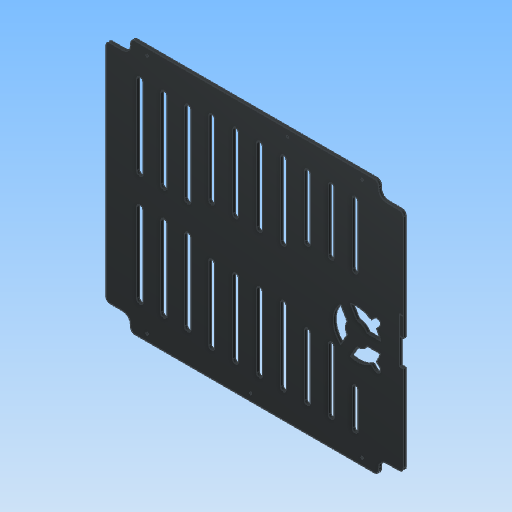
# Autodesk Inventor part: поддон1
Saved by Autodesk Inventor 2017 (Build 210142000, 142)
## iProperties
Part Number: поддон1
Material: Типовые
Document SubType Name: Modeling
Designer: Max
Density: 1 g/cm^3
Appearance: Чугун серый
Mass: 323.562 g
Surface Area: 2205.86 cm^2
Volume: 323.562 cm^3
Author: Max
Autodesk Inventor part; units mm, degrees
ref_plane "YZ Plane" through (0, 0, 0) normal (1, 0, 0) x (0, 1, 0)
ref_plane "XZ Plane" through (0, 0, 0) normal (0, 1, 0) x (-1, 0, 0)
ref_plane "XY Plane" through (0, 0, 0) normal (0, 0, 1) x (1, 0, 0)
sketch "Эскиз1" plane through (0, 0, 0) normal (0, 0, 1) x (1, 0, 0)
  line L0 (186.5, -159.5) -> (-186.5, -159.5)
  line L1 (-186.5, -159.5) -> (-186.5, 159.5)
  line L2 (-186.5, 159.5) -> (186.5, 159.5)
  line L3 (186.5, 159.5) -> (186.5, -159.5)
  line L4 (186.5, -159.5) -> (-186.5, 159.5) construction
  line L5 (-186.5, -159.5) -> (186.5, 159.5) construction
  circle A0 centre (-2.4493, 121.4084) radius 1.5 construction
  circle A1 centre (336.5507, 121.4084) radius 1.5 construction
  circle A2 centre (336.5507, 427.4084) radius 1.5 construction
  circle A3 centre (-2.4493, 427.4084) radius 1.5 construction
  arc A4 (348.5507, 300.4084) -> (346.5507, 298.4084) centre (348.5507, 298.4084) ccw construction
  line L6 (348.5507, 300.4084) -> (350.5507, 300.4084) construction
  arc A5 (350.5507, 300.4084) -> (350.5507, 305.4084) centre (350.5507, 302.9084) ccw construction
  line L7 (350.5507, 305.4084) -> (348.5507, 305.4084) construction
  arc A6 (346.5507, 307.4084) -> (348.5507, 305.4084) centre (348.5507, 307.4084) ccw construction
  line L8 (346.5507, 307.4084) -> (346.5507, 412.4084) construction
  line L9 (346.5507, 412.4084) -> (267.5507, 412.4084) construction
  arc A7 (265.5507, 414.4084) -> (267.5507, 412.4084) centre (267.5507, 414.4084) ccw construction
  line L10 (265.5507, 414.4084) -> (265.5507, 416.4084) construction
  arc A8 (265.5507, 416.4084) -> (250.5507, 416.4084) centre (258.0507, 416.4084) ccw construction
  line L11 (250.5507, 416.4084) -> (250.5507, 414.4084) construction
  arc A9 (248.5507, 412.4084) -> (250.5507, 414.4084) centre (248.5507, 414.4084) ccw construction
  line L12 (248.5507, 412.4084) -> (192.5507, 412.4084) construction
  arc A10 (190.5507, 414.4084) -> (192.5507, 412.4084) centre (192.5507, 414.4084) ccw construction
  line L13 (190.5507, 414.4084) -> (190.5507, 421.9084) construction
  arc A11 (190.5507, 421.9084) -> (188.5507, 423.9084) centre (188.5507, 421.9084) ccw construction
  line L14 (188.5507, 423.9084) -> (142.5507, 423.9084) construction
  arc A12 (142.5507, 423.9084) -> (140.5507, 421.9084) centre (142.5507, 421.9084) ccw construction
  line L15 (140.5507, 421.9084) -> (140.5507, 414.4084) construction
  arc A13 (138.5507, 412.4084) -> (140.5507, 414.4084) centre (138.5507, 414.4084) ccw construction
  line L16 (138.5507, 412.4084) -> (82.5507, 412.4084) construction
  arc A14 (80.5507, 414.4084) -> (82.5507, 412.4084) centre (82.5507, 414.4084) ccw construction
  line L17 (80.5507, 414.4084) -> (80.5507, 416.4084) construction
  arc A15 (80.5507, 416.4084) -> (65.5507, 416.4084) centre (73.0507, 416.4084) ccw construction
  line L18 (65.5507, 416.4084) -> (65.5507, 414.4084) construction
  arc A16 (63.5507, 412.4084) -> (65.5507, 414.4084) centre (63.5507, 414.4084) ccw construction
  line L19 (63.5507, 412.4084) -> (-15.4493, 412.4084) construction
  line L20 (-15.4493, 412.4084) -> (-15.4493, 136.4084) construction
  line L21 (-15.4493, 136.4084) -> (92.5507, 136.4084) construction
  arc A17 (94.5507, 134.4084) -> (92.5507, 136.4084) centre (92.5507, 134.4084) ccw construction
  line L22 (94.5507, 134.4084) -> (94.5507, 122.4084) construction
  arc A18 (94.5507, 122.4084) -> (96.5507, 120.4084) centre (96.5507, 122.4084) ccw construction
  line L23 (96.5507, 120.4084) -> (127.5507, 120.4084) construction
  arc A19 (127.5507, 120.4084) -> (129.5507, 122.4084) centre (127.5507, 122.4084) ccw construction
  line L24 (129.5507, 122.4084) -> (129.5507, 134.4084) construction
  arc A20 (131.5507, 136.4084) -> (129.5507, 134.4084) centre (131.5507, 134.4084) ccw construction
  line L25 (131.5507, 136.4084) -> (164.5507, 136.4084) construction
  arc A21 (166.5507, 134.4084) -> (164.5507, 136.4084) centre (164.5507, 134.4084) ccw construction
  line L26 (166.5507, 134.4084) -> (166.5507, 119.4084) construction
  arc A22 (166.5507, 119.4084) -> (168.5507, 117.4084) centre (168.5507, 119.4084) ccw construction
  line L27 (168.5507, 117.4084) -> (289.5507, 117.4084) construction
  arc A23 (289.5507, 117.4084) -> (291.5507, 119.4084) centre (289.5507, 119.4084) ccw construction
  line L28 (291.5507, 119.4084) -> (291.5507, 134.4084) construction
  arc A24 (293.5507, 136.4084) -> (291.5507, 134.4084) centre (293.5507, 134.4084) ccw construction
  line L29 (293.5507, 136.4084) -> (346.5507, 136.4084) construction
  line L30 (346.5507, 136.4084) -> (346.5507, 196.4084) construction
  arc A25 (348.5507, 198.4084) -> (346.5507, 196.4084) centre (348.5507, 196.4084) ccw construction
  line L31 (348.5507, 198.4084) -> (350.5507, 198.4084) construction
  arc A26 (350.5507, 198.4084) -> (350.5507, 203.4084) centre (350.5507, 200.9084) ccw construction
  line L32 (350.5507, 203.4084) -> (348.5507, 203.4084) construction
  arc A27 (346.5507, 205.4084) -> (348.5507, 203.4084) centre (348.5507, 205.4084) ccw construction
  line L33 (346.5507, 205.4084) -> (346.5507, 298.4084) construction
  circle A28 centre (208.5507, 425.4084) radius 1.5 construction
  circle A29 centre (302.0507, 425.4084) radius 1.5 construction
  circle A30 centre (162.0507, 123.4084) radius 1.5 construction
  circle A31 centre (-2.4493, 427.4084) radius 1.5 construction
  circle A32 centre (336.5507, 121.4084) radius 1.5 construction
  circle A33 centre (351.5507, 272.4084) radius 1.5 construction
  circle A34 centre (351.5507, 252.4084) radius 1.5 construction
  circle A35 centre (-2.4493, 121.4084) radius 1.5 construction
  circle A36 centre (336.5507, 427.4084) radius 1.5 construction
  circle A37 centre (32.5507, 123.4084) radius 1.5 construction
  circle A38 centre (302.0507, 123.4084) radius 1.5 construction
  circle A39 centre (32.5507, 425.4084) radius 1.5 construction
  line L34 (-23.4493, 108.4084) -> (354.5507, 108.4084) construction
  line L35 (-23.4493, 440.4084) -> (-23.4493, 108.4084) construction
  line L36 (354.5507, 440.4084) -> (-23.4493, 440.4084) construction
  line L37 (354.5507, 108.4084) -> (354.5507, 440.4084) construction
  line L38 (134.75, 151) -> (-134.75, 151) construction
  line L39 (-134.75, 151) -> (-134.75, -151) construction
  line L40 (-134.75, -151) -> (134.75, -151) construction
  line L41 (134.75, -151) -> (134.75, 151) construction
  line L42 (134.75, 151) -> (-134.75, -151) construction
  line L43 (-134.75, 151) -> (134.75, -151) construction
  circle A40 centre (-134.75, -151) radius 1.5
  circle A41 centre (134.75, -151) radius 1.5
  circle A42 centre (134.75, 151) radius 1.5
  circle A43 centre (-134.75, 151) radius 1.5
  point P0 (0, 0)
  dimension "d0" = 373
  dimension "d1" = 319
  dimension "d2" = 3
  dimension "d3" = 3
  dimension "d4" = 3
  dimension "d5" = 3
  dimension "d6" = 8.5
  dimension "d7" = 8.5
  dimension "d8" = 51.75
  dimension "d11" = 269.5
  dimension "d12" = 302
  constraints: 24 end point, 4 centre point, 4 coincident, 4 midpoint, 4 parallel, 2 horizontal, 2 perpendicular
  measures "d0" distance between parallel lines of L1 L3
  measures "d1" distance between parallel lines of L0 L2
  measures "d2" diameter of A40
  measures "d3" diameter of A41
  measures "d4" diameter of A42
  measures "d5" diameter of A43
  measures "d6" distance from line of L2 L38.end
  measures "d7" distance from line of L0 L39.end
  measures "d8" distance between parallel lines of L1 L39
  measures "d11" distance of L38.end L38.start
  measures "d12" distance between parallel lines of L38 L40
extrude "Выдавливание1" add sketch "Эскиз1" along normal blind 3.2
sketch "Эскиз2" plane through (0, 0, 0) normal (0, 0, -1) x (-1, 0, 0)
  arc A0 (-179.25, 24) -> (-181.25, 26) centre (-181.25, 24) ccw projected
  line L0 (-181.25, 26) -> (-183.25, 26) projected
  arc A1 (-183.25, 31) -> (-183.25, 26) centre (-183.25, 28.5) ccw projected
  line L1 (-183.25, 31) -> (-181.25, 31) projected
  arc A2 (-181.25, 31) -> (-179.25, 33) centre (-181.25, 33) ccw projected
  line L2 (-179.25, 33) -> (-179.25, 138) projected
  line L3 (-179.25, 138) -> (-100.25, 138) projected
  arc A3 (-100.25, 138) -> (-98.25, 140) centre (-100.25, 140) ccw projected
  line L4 (-98.25, 140) -> (-98.25, 142) projected
  arc A4 (-83.25, 142) -> (-98.25, 142) centre (-90.75, 142) ccw projected
  line L5 (-83.25, 142) -> (-83.25, 140) projected
  arc A5 (-83.25, 140) -> (-81.25, 138) centre (-81.25, 140) ccw projected
  line L6 (-81.25, 138) -> (-25.25, 138) projected
  arc A6 (-25.25, 138) -> (-23.25, 140) centre (-25.25, 140) ccw projected
  line L7 (-23.25, 140) -> (-23.25, 147.5) projected
  arc A7 (-21.25, 149.5) -> (-23.25, 147.5) centre (-21.25, 147.5) ccw projected
  line L8 (-21.25, 149.5) -> (24.75, 149.5) projected
  arc A8 (26.75, 147.5) -> (24.75, 149.5) centre (24.75, 147.5) ccw projected
  line L9 (26.75, 147.5) -> (26.75, 140) projected
  arc A9 (26.75, 140) -> (28.75, 138) centre (28.75, 140) ccw projected
  line L10 (28.75, 138) -> (84.75, 138) projected
  arc A10 (84.75, 138) -> (86.75, 140) centre (84.75, 140) ccw projected
  line L11 (86.75, 140) -> (86.75, 142) projected
  arc A11 (101.75, 142) -> (86.75, 142) centre (94.25, 142) ccw projected
  line L12 (101.75, 142) -> (101.75, 140) projected
  arc A12 (101.75, 140) -> (103.75, 138) centre (103.75, 140) ccw projected
  line L13 (103.75, 138) -> (182.75, 138) projected
  line L14 (182.75, 138) -> (182.75, -138) projected
  line L15 (182.75, -138) -> (74.75, -138) projected
  arc A13 (74.75, -138) -> (72.75, -140) centre (74.75, -140) ccw projected
  line L16 (72.75, -140) -> (72.75, -152) projected
  arc A14 (70.75, -154) -> (72.75, -152) centre (70.75, -152) ccw projected
  line L17 (70.75, -154) -> (39.75, -154) projected
  arc A15 (37.75, -152) -> (39.75, -154) centre (39.75, -152) ccw projected
  line L18 (37.75, -152) -> (37.75, -140) projected
  arc A16 (37.75, -140) -> (35.75, -138) centre (35.75, -140) ccw projected
  line L19 (35.75, -138) -> (2.75, -138) projected
  arc A17 (2.75, -138) -> (0.75, -140) centre (2.75, -140) ccw projected
  line L20 (0.75, -140) -> (0.75, -155) projected
  arc A18 (-1.25, -157) -> (0.75, -155) centre (-1.25, -155) ccw projected
  line L21 (-1.25, -157) -> (-122.25, -157) projected
  arc A19 (-124.25, -155) -> (-122.25, -157) centre (-122.25, -155) ccw projected
  line L22 (-124.25, -155) -> (-124.25, -140) projected
  arc A20 (-124.25, -140) -> (-126.25, -138) centre (-126.25, -140) ccw projected
  line L23 (-126.25, -138) -> (-179.25, -138) projected
  line L24 (-179.25, -138) -> (-179.25, -78) projected
  arc A21 (-179.25, -78) -> (-181.25, -76) centre (-181.25, -78) ccw projected
  line L25 (-181.25, -76) -> (-183.25, -76) projected
  arc A22 (-183.25, -71) -> (-183.25, -76) centre (-183.25, -73.5) ccw projected
  line L26 (-183.25, -71) -> (-181.25, -71) projected
  arc A23 (-181.25, -71) -> (-179.25, -69) centre (-181.25, -69) ccw projected
  line L27 (-179.25, -69) -> (-179.25, 24) projected
  circle A24 centre (-41.25, 151) radius 1.5 projected
  circle A25 centre (-134.75, 151) radius 1.5 projected
  circle A26 centre (5.25, -151) radius 1.5 projected
  circle A27 centre (169.75, 153) radius 1.5 projected
  circle A28 centre (-169.25, -153) radius 1.5 projected
  circle A29 centre (-184.25, -2) radius 1.5 projected
  circle A30 centre (-184.25, -22) radius 1.5 projected
  circle A31 centre (169.75, -153) radius 1.5 projected
  circle A32 centre (-169.25, 153) radius 1.5 projected
  circle A33 centre (134.75, -151) radius 1.5 projected
  circle A34 centre (-134.75, -151) radius 1.5 projected
  circle A35 centre (134.75, 151) radius 1.5 projected
  line L28 (190.75, -166) -> (-187.25, -166) projected
  line L29 (190.75, 166) -> (190.75, -166) projected
  line L30 (-187.25, 166) -> (190.75, 166) projected
  line L31 (-187.25, -166) -> (-187.25, 166) projected
  point P0 (0, 0)
extrude "Выдавливание2" cut sketch "Эскиз2" against normal blind 3.2 contours A24 | A25 | A26
sketch "Эскиз3" plane through (0, 0, 0) normal (0, 0, -1) x (-1, 0, 0)
  line L0 (186.5, 159.5) -> (186.5, -159.5) projected
  line L1 (186.5, -159.5) -> (155.5, -159.5)
  line L2 (155.5, -159.5) -> (155.5, -141.5)
  line L3 (155.5, -141.5) -> (186.5, -141.5)
  line L4 (186.5, -141.5) -> (186.5, -159.5)
  circle A0 centre (0, 0) radius 22.6044
  line L5 (-186.5, -159.5) -> (-186.5, 159.5) projected
  line L6 (-186.5, -159.5) -> (-155.5, -159.5)
  line L7 (-155.5, -159.5) -> (-155.5, -141.5)
  line L8 (-155.5, -141.5) -> (-186.5, -141.5)
  line L9 (-186.5, -141.5) -> (-186.5, -159.5)
  line L10 (-186.5, 159.5) -> (-155.5, 159.5)
  line L11 (-155.5, 159.5) -> (-155.5, 141.5)
  line L12 (-155.5, 141.5) -> (-186.5, 141.5)
  line L13 (-186.5, 141.5) -> (-186.5, 159.5)
  line L14 (186.5, 159.5) -> (155.5, 159.5)
  line L15 (155.5, 159.5) -> (155.5, 141.5)
  line L16 (155.5, 141.5) -> (186.5, 141.5)
  line L17 (186.5, 141.5) -> (186.5, 159.5)
  line L18 (-186.5, 2.5) -> (-181.5, 2.5)
  line L19 (-181.5, 2.5) -> (-181.5, -28.5)
  line L20 (-181.5, -28.5) -> (-186.5, -28.5)
  line L21 (-186.5, -28.5) -> (-186.5, 2.5)
  line L22 (-186.5, -159.5) -> (186.5, -159.5) projected
  line L23 (144, 119.5) -> (144, 19.5) construction
  line L24 (148, 119.5) -> (148, 19.5)
  line L25 (140, 19.5) -> (140, 119.5)
  arc A1 (148, 119.5) -> (140, 119.5) centre (144, 119.5) ccw
  arc A2 (140, 19.5) -> (148, 19.5) centre (144, 19.5) ccw
  line L26 (186.5, 159.5) -> (-186.5, 159.5) projected
  arc A3 (148, -19.5) -> (140, -19.5) centre (144, -19.5) ccw construction
  line L27 (140, -119.5) -> (140, -19.5) construction
  arc A4 (140, -119.5) -> (148, -119.5) centre (144, -119.5) ccw construction
  line L28 (148, -19.5) -> (148, -119.5) construction
  line L29 (144, -19.5) -> (144, -119.5) construction
  arc A5 (118, 119.5) -> (110, 119.5) centre (114, 119.5) ccw
  line L30 (110, 19.5) -> (110, 119.5)
  arc A6 (110, 19.5) -> (118, 19.5) centre (114, 19.5) ccw
  line L31 (118, 119.5) -> (118, 19.5)
  line L32 (114, 119.5) -> (114, 19.5) construction
  arc A7 (118, -19.5) -> (110, -19.5) centre (114, -19.5) ccw construction
  line L33 (110, -119.5) -> (110, -19.5) construction
  arc A8 (110, -119.5) -> (118, -119.5) centre (114, -119.5) ccw construction
  line L34 (118, -19.5) -> (118, -119.5) construction
  line L35 (114, -19.5) -> (114, -119.5) construction
  arc A9 (88, 119.5) -> (80, 119.5) centre (84, 119.5) ccw
  line L36 (80, 19.5) -> (80, 119.5)
  arc A10 (80, 19.5) -> (88, 19.5) centre (84, 19.5) ccw
  line L37 (88, 119.5) -> (88, 19.5)
  line L38 (84, 119.5) -> (84, 19.5) construction
  arc A11 (88, -19.5) -> (80, -19.5) centre (84, -19.5) ccw construction
  line L39 (80, -119.5) -> (80, -19.5) construction
  arc A12 (80, -119.5) -> (88, -119.5) centre (84, -119.5) ccw construction
  line L40 (88, -19.5) -> (88, -119.5) construction
  line L41 (84, -19.5) -> (84, -119.5) construction
  line L42 (54, 125) -> (54, 33) construction
  line L43 (57.5, 125) -> (57.5, 33)
  line L44 (50.5, 33) -> (50.5, 125)
  arc A13 (57.5, 125) -> (50.5, 125) centre (54, 125) ccw
  arc A14 (50.5, 33) -> (57.5, 33) centre (54, 33) ccw
  line L45 (0, 0) -> (241.9404, 0) construction
  line L46 (20.5, 33) -> (20.5, 125)
  arc A15 (27.5, 125) -> (20.5, 125) centre (24, 125) ccw
  line L47 (27.5, 125) -> (27.5, 33)
  arc A16 (20.5, 33) -> (27.5, 33) centre (24, 33) ccw
  line L48 (-9.5, 33) -> (-9.5, 125)
  arc A17 (-2.5, 125) -> (-9.5, 125) centre (-6, 125) ccw
  line L49 (-2.5, 125) -> (-2.5, 33)
  arc A18 (-9.5, 33) -> (-2.5, 33) centre (-6, 33) ccw
  line L50 (-39.5, 33) -> (-39.5, 125)
  arc A19 (-32.5, 125) -> (-39.5, 125) centre (-36, 125) ccw
  line L51 (-32.5, 125) -> (-32.5, 33)
  arc A20 (-39.5, 33) -> (-32.5, 33) centre (-36, 33) ccw
  line L52 (-66, 125) -> (-66, 48) construction
  line L53 (-62.5, 125) -> (-62.5, 48)
  line L54 (-69.5, 48) -> (-69.5, 125)
  arc A21 (-62.5, 125) -> (-69.5, 125) centre (-66, 125) ccw
  arc A22 (-69.5, 48) -> (-62.5, 48) centre (-66, 48) ccw
  line L55 (-36, 125) -> (-124.3885, 125) construction
  arc A23 (-92.5, 125) -> (-99.5, 125) centre (-96, 125) ccw
  line L56 (-92.5, 125) -> (-92.5, 48)
  line L57 (-96, 125) -> (-96, 48) construction
  line L58 (-99.5, 48) -> (-99.5, 125)
  arc A24 (-99.5, 48) -> (-92.5, 48) centre (-96, 48) ccw
  arc A25 (-122.5, 125) -> (-129.5, 125) centre (-126, 125) ccw
  line L59 (-122.5, 125) -> (-122.5, 48)
  line L60 (-126, 125) -> (-126, 48) construction
  line L61 (-129.5, 48) -> (-129.5, 125)
  arc A26 (-129.5, 48) -> (-122.5, 48) centre (-126, 48) ccw
  line L62 (0, 0) -> (267.6942, 0) construction
  point P0 (144, 69.5)
  point P1 (144, -69.5)
  point P2 (114, 69.5)
  point P3 (114, -69.5)
  point P4 (84, 69.5)
  point P5 (84, -69.5)
  point P6 (54, 79)
  point P7 (-66, 86.5)
  point P8 (-96, 86.5)
  point P9 (-126, 86.5)
  dimension "d15" = 18
  dimension "d16" = 31
  dimension "d17" = 18
  dimension "d18" = 31
  dimension "d19" = 18
  dimension "d20" = 31
  dimension "d21" = 131
  dimension "d22" = 162
  dimension "d23" = 5
  dimension "d24" = 8
  dimension "d25" = 108
  dimension "d26" = 46.5
  dimension "d27" = 36
  dimension "d30" = 139
  dimension "d33" = 30
  dimension "d36" = 38
  dimension "d37" = 31
  dimension "d38" = 19.5
  dimension "d39" = 19.5
  dimension "d40" = 30
  dimension "d41" = 7
  dimension "d42" = 99
  dimension "d43" = 31
  dimension "d46" = 30
  dimension "d51" = 7
  dimension "d52" = 84
  dimension "d53" = 30
  dimension "d56" = 30
  constraints: 138 end point, 52 point on circle, 27 centre point, 13 parallel, 12 tangent, 11 horizontal, 5 perpendicular, 4 point on line, 4 vertical, 3 midpoint, 1 coincident, 1 collinear, 113 other
  measures "d15" distance between parallel lines of L1 L3
  measures "d16" distance between parallel lines of L2 L0
  measures "d17" distance between parallel lines of L8 L6
  measures "d18" distance between parallel lines of L5 L7
  measures "d19" distance between parallel lines of L10 L12
  measures "d20" distance between parallel lines of L0 L15
  measures "d21" distance between parallel lines of L22 L20
  measures "d22" distance between parallel lines of L22 L18
  measures "d23" distance between parallel lines of L21 L19
  measures "d24" distance between parallel lines of L25 L24
  measures "d26" distance between parallel lines of L0 L25
  measures "d27" distance edge to line of A1 L26
  measures "d30" distance of L25.end L27.end
  measures "d33" distance of L25.end L30.end
  measures "d36" distance between parallel lines of L24 L30
  measures "d38" vertical distance of L23.end point (0, 0)
  measures "d39" vertical distance of point (0, 0) L29.start
  measures "d40" distance between parallel lines of L38 L42
  measures "d41" distance between parallel lines of L43 L44
  measures "d43" distance edge to line of A13 L26
  measures "d46" distance of L44.start L46.start
  measures "d51" distance between parallel lines of L53 L54
  measures "d53" distance from line of L55.start L52
  measures "d56" distance of L53.start L56.start
extrude "Выдавливание3" cut sketch "Эскиз3" against normal blind 3.2 contours L0 L16 L15 L14 | L0 L1 L2 L3 | L11 L12 L5 L10 | L6 L5 L8 L7 | L18 L19 L20 L5 | L24 A2 L25 A1 | L31 A6 L30 A5 | L37 A10 L36 A9 | L43 A14 L44 A13 | L46 A15 L47 A16 | L48 A17 L49 A18 | L50 A19 L51 A20 | L53 A22 L54 A21 | L56 A24 L58 A23 | L59 A26 L61 A25
fillet "Сопряжение1" radius 5 12 edges at (-155.5, 141.5, 1.6) (-155.5, 159.5, 1.6) (-186.5, 141.5, 1.6) (155.5, 159.5, 1.6) (155.5, 141.5, 1.6) (186.5, 141.5, 1.6) (155.5, -141.5, 1.6) (186.5, -141.5, 1.6) (155.5, -159.5, 1.6) (-155.5, -159.5, 1.6) (-155.5, -141.5, 1.6) (-186.5, -141.5, 1.6)
mirror "Зеркальное отражение1" about plane through (0, 0, 0) normal (0, 1, 0) of "Выдавливание3"
fillet "Сопряжение2" radius 10 4 edges at (-155.5, -141.5, 1.6) (-155.5, 141.5, 1.6) (155.5, 141.5, 1.6) (155.5, -141.5, 1.6)
sketch "Эскиз4" plane through (0, 0, 0) normal (0, 0, -1) x (-1, 0, 0)
  circle A0 centre (-128.5, -19.5) radius 30
  line L0 (-186.5, -28.5) -> (-186.5, -136.5) projected
  line L1 (-150.5, -159.5) -> (150.5, -159.5) projected
  line L2 (-128.5, -19.5) -> (-227.6748, -19.5) construction
  line L3 (-128.5, -19.5) -> (-153.6023, 5.6023) construction
  line L4 (-153.6023, 5.6023) -> (-153.6023, -44.6023) construction
  line L5 (-153.6023, -44.6023) -> (-128.5, -19.5) construction
  circle A1 centre (-153.6023, 5.6023) radius 4.5
  circle A2 centre (-153.6023, -44.6023) radius 4.5
  line L6 (-156.7843, 2.4203) -> (-152.6552, -1.7088)
  line L7 (-156.7843, 2.4203) -> (-150.4203, 8.7843)
  line L8 (-150.4203, 8.7843) -> (-146.2912, 4.6552)
  line L9 (-153.6023, -44.6023) -> (-156.7843, -41.4203)
  line L10 (-156.7843, -41.4203) -> (-152.6552, -37.2912)
  line L11 (-153.6023, -44.6023) -> (-150.4203, -47.7843)
  line L12 (-150.4203, -47.7843) -> (-146.2912, -43.6552)
  circle A3 centre (-128.5, -19.5) radius 14.5
  line L13 (-141.1984, -12.5) -> (-157.6719, -12.5)
  line L14 (-141.1984, -26.5) -> (-157.6719, -26.5)
  line L15 (-128.5, -19.5) -> (-113.5, -45.4808) construction
  line L16 (-128.5, -19.5) -> (-113.5, 6.4808) construction
  line L17 (-128.213, -33.9972) -> (-119.9762, -48.2636)
  line L18 (-116.0886, -26.9972) -> (-107.8519, -41.2636)
  line L19 (-116.0886, -12.0028) -> (-107.8519, 2.2636)
  line L20 (-128.213, -5.0028) -> (-119.9762, 9.2636)
  point P0 (0, 0)
  dimension "d65" = 60
  dimension "d66" = 58
  dimension "d67" = 140
  dimension "d71" = 90
  dimension "d72" = 9
  dimension "d73" = 9
  dimension "d74" = 10
  dimension "d75" = 10
  dimension "d76" = 29
  dimension "d77" = 120
  dimension "d78" = 120
  dimension "d79" = 120
  dimension "d80" = 14
  dimension "d81" = 14
  dimension "d82" = 14
  constraints: 38 end point, 10 point on circle, 7 parallel, 5 perpendicular, 4 coincident, 3 centre point, 3 tangent, 1 horizontal, 1 point on line, 1 vertical, 21 other
  measures "d66" distance from line of L0 L2.start
  measures "d67" distance from line of L1 L2.start
  measures "d71" angle of L5 L3
  measures "d72" diameter of A1
  measures "d73" diameter of A2
  measures "d76" diameter of A3
  measures "d77" angle of L16 L2
  measures "d78" angle of L2 L15
  measures "d79" angle of L16 L15
  measures "d80" distance between parallel lines of L19 L20
  measures "d81" distance between parallel lines of L17 L18
  measures "d82" distance between parallel lines of L14 L13
sketch "Эскиз5" plane through (0, 0, 0) normal (0, 0, -1) x (-1, 0, 0)
  line L0 (-122.5, -48) -> (-122.5, -125) projected
  arc A0 (-122.5, -48) -> (-129.5, -48) centre (-126, -48) ccw projected
  line L1 (-129.5, -125) -> (-129.5, -48) projected
  arc A1 (-129.5, -125) -> (-122.5, -125) centre (-126, -125) ccw projected
  line L2 (-126, -125) -> (-126, -80) construction
  line L3 (-129.5, -48) -> (-129.5, -125) projected
  line L4 (-122.5, -125) -> (-122.5, -80)
  line L5 (-129.5, -80) -> (-129.5, -125)
  arc A2 (-129.5, -125) -> (-122.5, -125) centre (-126, -125) ccw
  arc A3 (-122.5, -80) -> (-129.5, -80) centre (-126, -80) ccw
  arc A4 (-122.5, -48) -> (-129.5, -48) centre (-126, -48) ccw projected
  line L6 (-129.5, -80) -> (-129.5, -48)
  line L7 (-122.5, -125) -> (-122.5, -48) projected
  line L8 (-129.5, -48) -> (-122.5, -48)
  line L9 (-122.5, -48) -> (-122.5, -80)
  point P0 (0, 0)
  point P1 (-126, -102.5)
  dimension "d68" = 52
  constraints: 14 end point, 5 tangent, 4 point on circle, 2 centre point, 2 parallel, 2 perpendicular, 1 midpoint, 1 vertical
extrude "Выдавливание4" add sketch "Эскиз5" against normal blind 3.2 contours L8 A0 | L0 A3 L1 L8
extrude "Выдавливание5" cut sketch "Эскиз4" against normal blind 3.2 contours A0 L18 A3 L19 | L20 A3 L13 A0 | A0 L14 A3 L17 | A0 L6 A1 L8 | L12 A2 L10 A0 | L7 A1 | A1 L7 | L11 L9 A2 | A2 L9 L11
sketch "Эскиз7" plane through (0, 0, 0) normal (0, 0, -1) x (-1, 0, 0)
  line L0 (-186.5, 28.5) -> (-181.5, 28.5) projected
  line L1 (-181.5, -28.5) -> (-181.5, 28.5) projected
  line L2 (-186.5, 28.5) -> (-181.5, 28.5)
  line L3 (-181.5, 28.5) -> (-181.5, 4.5)
  line L4 (-181.5, 4.5) -> (-186.5, 4.5)
  line L5 (-186.5, 4.5) -> (-186.5, 28.5)
  line L6 (-181.5, -28.5) -> (-186.5, -28.5) projected
  point P0 (0, 0)
  dimension "d87" = 33
  constraints: 8 end point, 2 parallel, 1 horizontal, 1 perpendicular, 1 point on line
  measures "d87" distance between parallel lines of L4 L6
extrude "Выдавливание7" add sketch "Эскиз7" against normal blind 3
